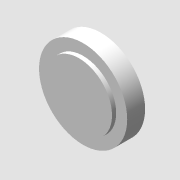
# Autodesk Inventor part: Wheel
Saved by Autodesk Inventor 2013 SP2 (Build 170200200, 200)
## iProperties
Created: 2014-04-23
Part Number: Wheel
Material: Generic
Document SubType Name: Modeling
Designer: Kevin
Density: 1 g/cm^3
Author: Kevin
Autodesk Inventor part; units mm, degrees
ref_plane "YZ Plane" through (0, 0, 0) normal (1, 0, 0) x (0, 1, 0)
ref_plane "XZ Plane" through (0, 0, 0) normal (0, 1, 0) x (-1, 0, 0)
ref_plane "XY Plane" through (0, 0, 0) normal (0, 0, 1) x (1, 0, 0)
sketch "Sketch1" plane through (0, 0, 0) normal (0, 0, 1) x (1, 0, 0)
  circle A0 centre (0, 0) radius 16
  dimension "d0" = 32
  constraints: 1 centre point, 1 coincident
  measures "d0" diameter of A0
extrude "Extrusion1" add sketch "Sketch1" against normal blind 9
sketch "Sketch2" plane through (0, 0, 0) normal (0, 0, 1) x (1, 0, 0)
  circle A0 centre (0, 0) radius 16 projected
  circle A1 centre (0, 0) radius 16
  circle A2 centre (0, 0) radius 12
  dimension "d3" = 32
  dimension "d4" = 24
  constraints: 2 centre point, 2 coincident
  measures "d3" diameter of A1
  measures "d4" diameter of A2
extrude "Extrusion2" cut sketch "Sketch2" against normal blind 1.5
sketch "Sketch3" plane through (0, 0, 0) normal (0, 0, 1) x (1, 0, 0)
  circle A0 centre (0, 0) radius 12 projected
  arc A1 (-1.118, 1) -> (1.118, 1) centre (0, 0) ccw
  line L0 (0, 0) -> (0, 1)
  line L1 (0, 1) -> (-1.118, 1)
  line L2 (0, 1) -> (1.118, 1)
  arc A2 (1.118, 1) -> (-1.118, 1) centre (0, 0) ccw
  dimension "d7" = 3
  dimension "d8" = 1
  constraints: 6 end point, 4 point on circle, 2 centre point, 1 coincident, 1 collinear, 1 perpendicular, 1 vertical
  measures "d7" diameter of A1
  measures "d8" distance of L0.start L0.end
extrude "Extrusion3" cut sketch "Sketch3" against normal blind 8 contours L1 L2 A1
body "Solid1"
